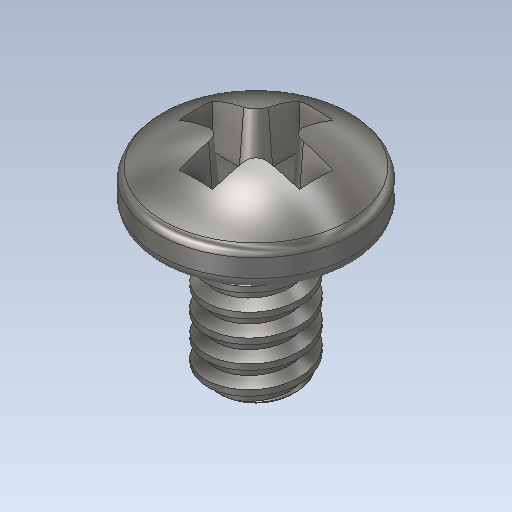
# Autodesk Inventor part: 91772A349
Saved by Autodesk Inventor 2020 (Build 240168000, 168)
## iProperties
Created: 2018-09-02
Part Number: 91772A349
Material: Stainless Steel
Document SubType Name: Modeling
Designer: amsmi
Density: 8 g/cm^3
Appearance: Semi-Polished
Mass: 0.468326 g
Surface Area: 1.51203 cm^2
Volume: 0.0585408 cm^3
Catalog Web Link: www.mcmaster.com/#91772A349
Author: amsmi
Autodesk Inventor part; units mm, degrees
ref_plane "YZ Plane" through (0, 0, 0) normal (1, 0, 0) x (0, 1, 0)
ref_plane "XZ Plane" through (0, 0, 0) normal (0, 1, 0) x (-1, 0, 0)
sketch "Sketch1" plane through (0, 0, 0) normal (0, 0, 1) x (1, 0, 0)
  line L0 (0, 0) -> (1.0116, 0)
  line L1 (1.0116, 0) -> (1.3291, 0.3175)
  line L2 (1.3291, 0.3175) -> (1.3291, 3.9688)
  line L3 (1.3291, 3.9688) -> (2.4367, 3.9687)
  arc A0 (2.4367, 3.9687) -> (2.7813, 4.3133) centre (2.4367, 4.3133) ccw
  line L4 (2.7813, 4.3133) -> (2.7813, 4.8213)
  arc A1 (2.7813, 4.8213) -> (2.648, 5.0935) centre (2.4367, 4.8213) ccw
  arc A2 (2.648, 5.0935) -> (0, 6.0008) centre (0, 1.6828) ccw
  line L5 (0, 0) -> (0, 6.0008)
  line L6 (0, 6.0008) -> (0, -1.9367)
  dimension "d0" = 2.032
  dimension "d2" = 45
  dimension "d3" = 0.3175
  dimension "d4" = 2.6581
  dimension "d5" = 5.5626
  dimension "d6" = 0.508
  dimension "d8" = 4.318
  dimension "d9" = 3.9688
  dimension "d11" = 7.9375
  constraints: 14 end point, 6 point on circle, 4 tangent, 3 centre point, 2 horizontal, 2 horizontal alignment, 2 perpendicular, 2 vertical, 1 equal radius, 1 line through centre
  measures "d0" distance from line of L3 L5.end
  measures "d2" angle of L0 L1
  measures "d3" horizontal distance of L0.end L1.end
  measures "d4" diameter of L2 L6
  measures "d5" diameter of L4 L6
  measures "d6" distance of L4.start L4.end
  measures "d8" radius of A2
  measures "d9" distance between parallel lines of L0 L3
  measures "d11" distance of L5.end L6.end
revolve "Revolution1" add sketch "Sketch1" angle 360 about axis through (0, 6.0008, 0) along (0, -1, 0)
sketch "Sketch2" plane through (0, 0, 0) normal (1, 0, 0) x (0, 1, 0)
  line L0 (4.445, -1.3291) -> (3.9688, -1.3291)
  line L1 (3.9688, -1.3291) -> (4.1275, -1.0541)
  line L2 (4.1275, -1.0541) -> (4.2862, -1.0541)
  line L3 (4.2862, -1.0541) -> (4.445, -1.3291)
  line L4 (0.3175, -1.3291) -> (3.9688, -1.3291) construction
  point P0 (0, 0)
  dimension "d12" = 60
  dimension "d13" = 0.4763
  dimension "d14" = 0.1588
  constraints: 8 end point, 1 equal length, 1 horizontal, 1 parallel
  measures "d12" angle of L1 L3
  measures "d13" distance of L0.end L0.start
  measures "d14" distance of L1.end L2.end
coil "Coil1" sketch "Sketch2" operation cut axis through (0, -10, 0) along (0, -1, 0) pitch 0.635 turns 7.75 hand right
sketch "Sketch3" plane through (0, 3.9687, 0) normal (0, -1, 0) x (1, 0, 0)
  circle A0 centre (0, 0) radius 2.4367 projected
  line L0 (0, 0) -> (-1016, 0) construction
  line L1 (0, 0) -> (0, -101.6) construction
  point P0 (0, 0)
  dimension "d45" = 1016
  dimension "d46" = 101.6
  constraints: 4 end point, 1 horizontal, 1 vertical
  measures "d45" distance of L0.start L0.end
  measures "d46" distance of L0.start L1.end
extrude "Extrusion1" add sketch "Sketch3" against normal up to surface
ref_plane "Work Plane1" through (0, 6.0008, 0) normal (0, -1, 0) x (1, 0, 0)
sketch "Sketch6" plane through (0, 6.0008, 0) normal (0, -1, 0) x (1, 0, 0)
  line L0 (-0.508, 1.7383) -> (0.508, 1.7383)
  line L1 (0.508, -1.7383) -> (-0.508, -1.7383)
  line L2 (1.7383, 0.508) -> (1.7383, -0.508)
  line L3 (-1.7383, -0.508) -> (-1.7383, 0.508)
  arc A0 (-0.8467, 0.508) -> (-0.508, 0.8467) centre (-0.8467, 0.8467) ccw
  arc A1 (-0.508, -0.8467) -> (-0.8467, -0.508) centre (-0.8467, -0.8467) ccw
  arc A2 (0.508, 0.8467) -> (0.8467, 0.508) centre (0.8467, 0.8467) ccw
  arc A3 (0.8467, -0.508) -> (0.508, -0.8467) centre (0.8467, -0.8467) ccw
  line L4 (-1.7383, 0.508) -> (-0.8467, 0.508)
  line L5 (0.8467, 0.508) -> (1.7383, 0.508)
  line L6 (-0.508, -1.7383) -> (-0.508, -0.8467)
  line L7 (-0.508, 0.8467) -> (-0.508, 1.7383)
  line L8 (0.508, 1.7383) -> (0.508, 0.8467)
  line L9 (0.508, -0.8467) -> (0.508, -1.7383)
  line L10 (1.7383, -0.508) -> (0.8467, -0.508)
  line L11 (-0.8467, -0.508) -> (-1.7383, -0.508)
  point P0 (0, 0)
  point P1 (0, 1.7383)
  point P2 (-1.7383, 0)
  dimension "d40" = 3.4766
  dimension "d41" = 1.016
  dimension "d42" = 0.3387
  constraints: 24 end point, 16 tangent, 10 parallel, 8 point on circle, 4 centre point, 4 equal length, 4 perpendicular, 3 equal radius, 3 horizontal, 2 midpoint, 1 horizontal alignment, 1 vertical alignment
  measures "d40" distance between parallel lines of L2 L3
  measures "d41" distance of L1.start L1.end
  measures "d42" radius of A3
extrude "Extrusion3" cut sketch "Sketch6" along normal blind 1.524 draft -5
equation "\"d0\" = HeadHeight"
equation "\"d3\" = 0.5 * Pitch"
equation "\"d4\" = MajorDia"
equation "\"d5\" = HeadDia"
equation "\"d6\" = 0.25 * d0"
equation "\"d8\" = 0.776256 * d5"
equation "\"d9\" = Length"
equation "\"d11\" = 2 * Length"
equation "\"d13\" = 0.75 * Pitch"
equation "\"d14\" = 0.25 * Pitch"
equation "\"d15\" = Pitch"
equation "\"d16\" = Length + 1.5 * Pitch"
equation "\"d45\" = 25.4 * TPI"
equation "\"d46\" = 25.4 * Gauge"
equation "\"d40\" = 0.625 * HeadDia"
equation "\"d41\" = 0.5 * HeadHeight"
equation "\"d42\" = 0.333333 * d41"
equation "\"d43\" = 0.75 * HeadHeight"
equation "\"Length\" = 3.96875"
equation "\"MajorDia\" = 2.65813"
equation "\"HeadDia\" = 5.5626"
equation "\"HeadHeight\" = 2.032"
equation "\"Pitch\" = 0.635"
equation "\"TPI\" = 40"
equation "\"Gauge\" = 4"
body "Solid1"
